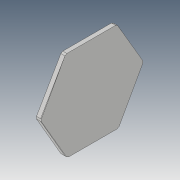
# Autodesk Inventor part: cordGripGasket
Saved by Autodesk Inventor 2018 (Build 220112000, 112)
## iProperties
Created: 2020-03-11
Part Number: cordGripGasket
Material: Generic
Document SubType Name: Modeling
Designer: anirudh
Density: 1 g/cm^3
Appearance: Default
Author: anirudh
Autodesk Inventor part; units mm, degrees
ref_plane "YZ Plane" through (0, 0, 0) normal (1, 0, 0) x (0, 1, 0)
ref_plane "XZ Plane" through (0, 0, 0) normal (0, 1, 0) x (-1, 0, 0)
ref_plane "XY Plane" through (0, 0, 0) normal (0, 0, 1) x (1, 0, 0)
sketch "Sketch1" plane through (0, 0, 0) normal (1, 0, 0) x (0, 1, 0)
  arc A0 (-10.7802, 6.2239) -> (-10.922, 5.9782) centre (-5.461, 2.9891) ccw
  line L0 (-10.7802, 6.2239) -> (-10.922, 5.9782)
  arc A1 (-10.922, 0) -> (-10.7802, -0.2457) centre (-5.461, 2.9891) ccw
  line L1 (-10.922, 5.9782) -> (-10.922, 0)
  line L2 (-10.7802, -0.2457) -> (-5.6028, -3.2348)
  line L3 (-10.922, 0) -> (-10.7802, -0.2457)
  line L4 (-10.7802, -0.2457) -> (-5.6028, -3.2348)
  line L5 (-0.1418, -0.2457) -> (-5.3192, -3.2348)
  line L6 (-5.6028, -3.2348) -> (-5.3192, -3.2348)
  line L7 (-5.3192, -3.2348) -> (-0.1418, -0.2457)
  arc A2 (-0.1418, -0.2457) -> (0, 0) centre (-5.461, 2.9891) ccw
  line L8 (-0.1418, -0.2457) -> (-0.1418, -0.2457)
  line L9 (-0.1418, -0.2457) -> (0, 0)
  line L10 (0, 0) -> (0, 5.9782)
  line L11 (0, 0) -> (0, 5.9782)
  line L12 (-5.3192, 9.213) -> (-0.1418, 6.2239)
  line L13 (0, 5.9782) -> (-0.1418, 6.2239)
  line L14 (-0.1418, 6.2239) -> (-5.3192, 9.213)
  line L15 (-5.6028, 9.213) -> (-10.7802, 6.2239)
  line L16 (-5.3192, 9.213) -> (-5.6028, 9.213)
  line L17 (-5.6028, 9.213) -> (-10.7802, 6.2239)
  line L18 (0, 2.9891) -> (0, -8.0007)
  constraints: 38 end point, 6 point on circle, 4 collinear, 3 centre point, 2 perpendicular, 2 vertical, 1 midpoint, 1 point on line, 1 tangent
extrude "Extrusion1" add sketch "Sketch1" along normal blind 0.5
sketch "Sketch2" plane through (0.5, 0, 0) normal (1, 0, 0) x (0, 0, -1)
  line L0 (-9.213, -5.6028) -> (-6.2239, -10.7802) projected
  line L1 (3.2348, -5.3192) -> (0.2457, -0.1418) projected
  line L2 (-6.2239, -10.7802) -> (-5.9782, -10.922)
  line L3 (-9.213, -5.3192) -> (-9.213, -5.6028)
  line L4 (-6.2239, -10.7802) -> (-9.213, -5.6028)
  line L5 (-9.213, -5.6028) -> (-6.2239, -10.7802)
  line L6 (-5.9782, -10.922) -> (0, -10.922)
  line L7 (-5.9782, -10.922) -> (0, -10.922)
  line L8 (-6.2239, -0.1418) -> (-9.213, -5.3192)
  line L9 (-6.2239, -0.1418) -> (-9.213, -5.3192)
  line L10 (-5.9782, 0) -> (-6.2239, -0.1418)
  arc A0 (-5.9782, 0) -> (-6.2239, -0.1418) centre (-2.9891, -5.461) ccw
  line L11 (-5.9782, 0) -> (-5.9782, 0)
  line L12 (-5.9782, 0) -> (0, 0)
  line L13 (0, 0) -> (-5.9782, 0)
  line L14 (0, -10.922) -> (0.2457, -10.7802)
  arc A1 (0, -10.922) -> (0.2457, -10.7802) centre (-2.9891, -5.461) ccw
  line L15 (0.2457, -10.7802) -> (3.2348, -5.6028)
  line L16 (0.2457, -0.1418) -> (0, 0)
  line L17 (3.2348, -5.6028) -> (3.2348, -5.3192)
  line L18 (3.2348, -5.3192) -> (0.2457, -0.1418)
  line L19 (3.2348, -5.3192) -> (0.2457, -0.1418)
  arc A2 (3.2348, -5.6028) -> (3.2348, -5.3192) centre (-2.9891, -5.461) ccw
  line L20 (-2.9891, 0) -> (6.4696, 0)
  point P0 (-2.9891, -5.461)
  point P1 (-6.3658, 3.093)
  constraints: 38 end point, 6 point on circle, 4 collinear, 3 centre point, 2 perpendicular, 1 horizontal, 1 midpoint, 1 tangent
revolve "Revolution1" add sketch "Sketch2" angle 1 about axis through (0.5, 0, 2.9891) along (0, 0, 1)
body "Solid1"
